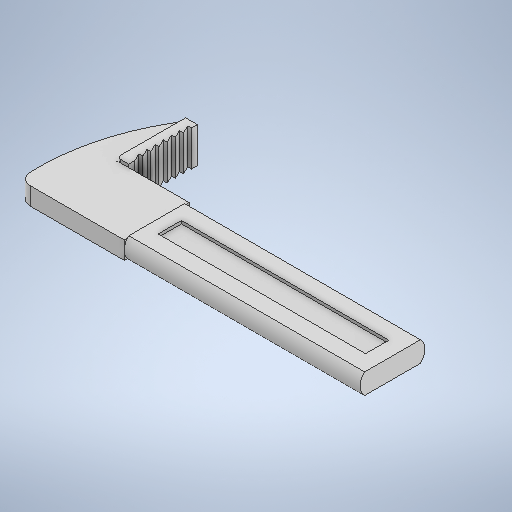
# Autodesk Inventor part: Top
Saved by Autodesk Inventor 2025.1 (Build 291241000, 241)
## iProperties
Created: 2024-08-16
Part Number: Top
Material: Generic
Document SubType Name: Modeling
Designer: vedan
Density: 1 g/cm^3
Appearance: Default
Author: vedan
Autodesk Inventor part; units mm, degrees
ref_plane "YZ Plane" through (0, 0, 0) normal (1, 0, 0) x (0, 1, 0)
ref_plane "XZ Plane" through (0, 0, 0) normal (0, 1, 0) x (-1, 0, 0)
ref_plane "XY Plane" through (0, 0, 0) normal (0, 0, 1) x (1, 0, 0)
sketch "Sketch1" plane through (0, 0, 0) normal (0, 1, 0) x (-1, 0, 0)
  line L0 (0, -131.5012) -> (-0.0617, -190.607)
  line L1 (-41.7658, -131.5012) -> (53.7037, -131.5012) construction
  line L2 (28.2495, -75.6212) -> (-41.7658, -75.6212)
  arc A0 (-0.0617, -190.607) -> (28.2495, -75.6212) centre (-152.8189, -92.0177) ccw
  line L3 (28.2495, -75.6212) -> (-62.1692, -75.6212)
  line L4 (-62.1692, -75.6212) -> (-62.1692, -131.5012)
  line L5 (-62.1692, -131.5012) -> (0, -131.5012)
  point P0 (0, 0)
  point P1 (8.9112, -179.6369)
  point P2 (0, -75.6212)
  point P3 (-70.1734, -131.5012)
  dimension "d21" = 59.1058
  dimension "d37" = 70.0153
  constraints: 12 end point, 3 horizontal, 2 point on circle, 1 centre point, 1 collinear, 1 perpendicular, 1 point on line
  measures "d21" distance of L0.start L0.end
  measures "d37" distance of L2.start L2.end
extrude "Extrusion1" add sketch "Sketch1" along normal blind 15.24
fillet "Fillet1" radius 10.16 1 edges at (-28.2495, 7.62, -75.6212)
sketch "Sketch4" plane through (0.0191, 12.7, -149.7788) normal (0.9999995, 0, 0.0010447) x (0.0010447, 0, -0.9999995)
  line L0 (0, -22.86) -> (0, 2.54)
  line L1 (15.9389, 2.54) -> (13.4561, 2.54) construction
  line L2 (13.4561, 2.54) -> (13.4561, 4.185) construction
  line L3 (13.6464, 2.54) -> (33.02, 2.54)
  line L4 (33.02, -22.86) -> (13.6464, -22.86)
  line L5 (-10.4713, -22.86) -> (-10.4713, 2.54) construction
  line L6 (-10.4713, -10.16) -> (33.02, -10.16) construction
  line L7 (-10.4713, -10.16) -> (11.2743, -10.16) construction
  line L8 (-18.2773, 5.1507) -> (40.826, 5.1507)
  line L9 (40.826, 5.1507) -> (40.826, -25.4707)
  line L10 (40.826, -25.4707) -> (-18.2773, -25.4707)
  line L11 (-18.2773, -25.4707) -> (-18.2773, 5.1507)
  line L12 (-18.2773, 5.1507) -> (40.826, -25.4707) construction
  line L13 (40.826, 5.1507) -> (-18.2773, -25.4707) construction
  point P0 (8.89, -10.16)
  dimension "d24" = 43.4913
  dimension "d23" = 21.7457
  constraints: 28 end point, 4 midpoint, 2 horizontal, 2 parallel, 1 perpendicular
  measures "d24" distance of L6.start L6.end
  measures "d23" distance of L6.start L7.end
extrude "Extrusion4" add sketch "Sketch4" along normal blind 10.16
sketch "Sketch5" plane through (0, 17.8507, -131.5015) normal (0, 1, 0) x (0.9999995, 0, 0.0010447)
  line L0 (10.16, 0) -> (10.16, 59.1033) projected
  line L1 (10.16, 0) -> (10.16, 4.6168)
  line L2 (10.16, 0) -> (10.16, 6.604)
  line L3 (10.16, 59.1033) -> (10.16, 54.0318)
  line L4 (10.16, 54.0318) -> (6.8983, 54.0318)
  line L5 (6.8983, 54.0318) -> (10.16, 47.0371)
  line L6 (10.16, 3.5366) -> (10.16, 0)
  line L7 (10.16, 54.0318) -> (10.16, 59.1033)
  line L8 (10.16, 47.0371) -> (6.8983, 47.0371)
  line L9 (6.8983, 47.0371) -> (10.16, 40.0424)
  line L10 (10.16, 40.0424) -> (6.8983, 40.0424)
  line L11 (6.8983, 40.0424) -> (10.16, 33.0478)
  line L12 (10.16, 33.0478) -> (6.8983, 33.0478)
  line L13 (6.8983, 33.0478) -> (10.16, 26.0531)
  line L14 (10.16, 26.0531) -> (6.8983, 26.0531)
  line L15 (6.8983, 26.0531) -> (10.16, 19.0584)
  line L16 (10.16, 19.0584) -> (6.8983, 19.0584)
  line L17 (6.8983, 19.0584) -> (10.16, 12.0637)
  line L18 (10.16, 12.0637) -> (6.8983, 12.0637)
  line L19 (6.8983, 12.0637) -> (10.16, 5.0691)
  line L20 (10.16, 5.0691) -> (10.16, 54.0318)
  point P0 (-241.3, 27.1673)
  dimension "d30" = 5.0715
  dimension "d28" = 65
  dimension "d29" = 6.9947
  constraints: 40 end point, 7 horizontal, 4 point on line, 2 collinear, 1 vertical
  measures "d30" distance of L0.end L3.end
  measures "d28" angle of L5 L4
  measures "d29" vertical distance of L4.end L5.end
extrude "Extrusion5" cut sketch "Sketch5" against normal through all
fillet "Fillet3" radius 3.175 1 edges at (0, 16.5453, -131.5015)
sketch "Sketch7" plane through (62.1692, 0, -75.6212) normal (1, 0, 0) x (0, 0, -1)
  line L0 (0, 15.24) -> (55.88, 15.24) projected
  line L1 (55.88, 0) -> (27.2823, 0)
  line L2 (27.94, 0) -> (41.91, 0) construction
  line L3 (55.88, 0) -> (55.88, 15.24) projected
  line L4 (55.88, 0) -> (27.94, 0)
  line L5 (9.7909, 0) -> (0, 0) projected
  line L6 (27.94, 0) -> (27.94, 15.24)
  line L7 (27.94, 15.24) -> (53.086, 15.24)
  line L8 (114.9858, 15.24) -> (9.7909, 15.24) projected
  arc A0 (51.9331, -1.1819) -> (51.9331, 16.4219) centre (44.0921, 7.62) ccw
  line L9 (51.9331, 16.4219) -> (51.9331, -1.1819) construction
  line L10 (51.9331, 16.4219) -> (69.5369, 16.4219) construction
  arc A1 (3.9469, 16.4219) -> (3.9469, -1.1819) centre (11.7879, 7.62) ccw
  line L11 (3.9469, 16.4219) -> (51.9331, 16.4219)
  line L12 (3.9469, -1.1819) -> (51.9331, -1.1819)
  point P0 (-75.6212, 0)
  dimension "d43" = 27.94
  dimension "d44" = 25.146
  dimension "d45" = 90
  dimension "d56" = 17.6038
  constraints: 18 end point, 4 point on circle, 3 symmetric about line, 2 centre point, 2 horizontal, 1 collinear, 1 midpoint, 1 perpendicular, 1 point on line, 1 other
  measures "d43" distance of L1.start L2.start
  measures "d44" distance of L6.end L7.end
  measures "d45" angle of L9 L10
  measures "d56" distance between parallel lines of L11 L12
extrude "Extrusion6" add sketch "Sketch7" along normal blind 203.2 contours L0 A1 L11 A0 | L0 L6 L1 A0 L12 A1 | L0 A0 L1 L6
sketch "Sketch8" plane through (62.1692, 16.4219, -79.5681) normal (0, 1, 0) x (1, 0, 0)
  line L0 (203.2, 47.9862) -> (203.2, 0) construction
  line L1 (203.2, 23.9931) -> (-91.0395, 23.9931) construction
  arc A0 (-62.1075, 111.0389) -> (-91.0395, 5.8439) centre (90.6496, 12.4496) ccw construction
  line L2 (-91.0395, 5.8439) -> (-91.0395, 27.6375) construction
  line L3 (-91.0395, 5.8439) -> (-69.2459, 5.8439) construction
  line L4 (203.2, 0) -> (56.0832, 0) construction
  line L5 (0, 0) -> (203.2, 0) construction
  line L6 (56.0832, 0) -> (56.0832, 60.6628) construction
  line L7 (-77.8013, 6.5731) -> (189.9677, 41.4131) construction
  line L8 (189.9677, 6.5731) -> (-77.8013, 41.4131) construction
  line L9 (11.3147, 13.9418) -> (189.9677, 13.9418)
  line L10 (189.9677, 13.9418) -> (189.9677, 34.0444)
  line L11 (189.9677, 34.0444) -> (11.3147, 34.0444)
  line L12 (11.3147, 34.0444) -> (11.3147, 13.9418)
  line L13 (11.3147, 13.9418) -> (189.9677, 34.0444) construction
  line L14 (189.9677, 13.9418) -> (11.3147, 34.0444) construction
  point P0 (-62.1692, -79.5681)
  point P1 (56.0832, 23.9931)
  point P2 (100.6412, 23.9931)
  dimension "d48" = 90
  dimension "d50" = 147.1168
  constraints: 26 end point, 5 midpoint, 4 point on line, 3 horizontal, 3 perpendicular, 2 parallel
  measures "d48" angle of L3 L2
  measures "d50" distance of L0.end L4.end
extrude "Extrusion7" cut sketch "Sketch8" against normal blind 2.54
body "Solid1"
